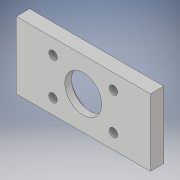
# Autodesk Inventor part: bottom_g2v1
Saved by Autodesk Inventor 2019 (Build 230136000, 136)
## iProperties
Created: 2018-08-27
Part Number: bottom_g2v1
Material: Generic
Document SubType Name: Modeling
Designer: Brian
Density: 1 g/cm^3
Appearance: Default
Author: Brian
Autodesk Inventor part; units mm, degrees
ref_plane "YZ Plane" through (0, 0, 0) normal (1, 0, 0) x (0, 1, 0)
ref_plane "XZ Plane" through (0, 0, 0) normal (0, 1, 0) x (-1, 0, 0)
ref_plane "XY Plane" through (0, 0, 0) normal (0, 0, 1) x (1, 0, 0)
sketch "Sketch1" plane through (0, 0, 0) normal (0, 0, 1) x (1, 0, 0)
  line L0 (0, 0) -> (40, 0)
  line L1 (40, 0) -> (40, 20)
  line L2 (40, 20) -> (0, 20)
  line L3 (0, 20) -> (0, 0)
  dimension "d0" = 40
  dimension "d1" = 20
  constraints: 8 end point, 2 parallel, 1 horizontal, 1 perpendicular
  measures "d0" distance of L2.end L1.end
  measures "d1" distance of L1.end L0.end
extrude "Extrusion1" add sketch "Sketch1" along normal blind 4
sketch "Sketch3" plane through (0, 0, 4) normal (0, 0, 1) x (1, 0, 0)
  line L0 (40, 20) -> (0, 20) projected
  line L1 (0, 20) -> (0, 0) projected
  point P0 (11, 15.5)
  dimension "d41" = 4.5
  dimension "d42" = 11
  measures "d41" distance from line of L0 point (11, 15.5)
  measures "d42" distance from line of L1 point (11, 15.5)
hole "Hole2" at (11, 15.5, 4) direction (0, 0, -1) diameter 2.5 end through all
sketch "Sketch4" plane through (0, 0, 4) normal (0, 0, 1) x (1, 0, 0)
  line L0 (0, 20) -> (0, 0) projected
  line L1 (0, 0) -> (40, 0) projected
  point P0 (11, 4.5)
  dimension "d43" = 11
  dimension "d44" = 4.5
  measures "d43" distance from line of L0 point (11, 4.5)
  measures "d44" distance from line of L1 point (11, 4.5)
hole "Hole3" at (11, 4.5, 4) direction (0, 0, -1) diameter 2.5 end through all
sketch "Sketch5" plane through (0, 0, 4) normal (0, 0, 1) x (1, 0, 0)
  line L0 (40, 0) -> (40, 20) projected
  line L1 (40, 20) -> (0, 20) projected
  point P0 (0, 0)
  point P1 (29, 15.5)
  dimension "d45" = 11
  dimension "d46" = 4.5
  measures "d45" distance from line of L0 point (29, 15.5)
  measures "d46" distance from line of L1 point (29, 15.5)
hole "Hole4" at (29, 15.5, 4) direction (0, 0, -1) diameter 2.5 end through all
sketch "Sketch6" plane through (0, 0, 4) normal (0, 0, 1) x (1, 0, 0)
  line L0 (40, 0) -> (40, 20) projected
  line L1 (0, 0) -> (40, 0) projected
  point P0 (29, 4.5)
  dimension "d47" = 11
  dimension "d48" = 4.5
  measures "d47" distance from line of L0 point (29, 4.5)
  measures "d48" distance from line of L1 point (29, 4.5)
hole "Hole5" at (29, 4.5, 4) direction (0, 0, -1) diameter 2.5 end through all
sketch "Sketch7" plane through (0, 0, 0) normal (0, 0, -1) x (-1, 0, 0)
  line L0 (0, 20) -> (0, 0) projected
  line L1 (-40, 20) -> (0, 20) projected
  point P0 (-19.9898, 9.9924)
  dimension "d56" = 19.9898
  dimension "d57" = 10.0076
  measures "d56" distance from line of L0 point (-19.99, 9.992)
  measures "d57" distance from line of L1 point (-19.99, 9.992)
hole "Hole6" at (19.9898, 9.9924, 0) direction (0, 0, 1) diameter 11 end through all counterbore diameter 16.2 counterbore depth 2
body "Solid1"
